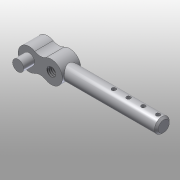
# Autodesk Inventor part: 500-178
Saved by Autodesk Inventor 2016 (Build 200138000, 138)
## iProperties
Created: 2015-04-18
Part Number: 500-178
Material: ABS Plastic
Document SubType Name: Modeling
Designer: Station9
Density: 1.06 g/cm^3
Appearance: Smooth - White
Mass: 0.63043 g
Surface Area: 6.93411 cm^2
Volume: 0.594746 cm^3
Author: Station9
Autodesk Inventor part; units mm, degrees
ref_plane "YZ Plane" through (0, 0, 0) normal (1, 0, 0) x (0, 1, 0)
ref_plane "XZ Plane" through (0, 0, 0) normal (0, 1, 0) x (-1, 0, 0)
ref_plane "XY Plane" through (0, 0, 0) normal (0, 0, 1) x (1, 0, 0)
sketch "Sketch1" plane through (0, 0, 0) normal (0, 1, 0) x (-1, 0, 0)
  arc A0 (1.5, -2.5981) -> (1.5, 2.5981) centre (3, 0) ccw
  arc A1 (-1.5, 2.5981) -> (-1.5, -2.5981) centre (-3, 0) ccw
  arc A2 (-1.5, 2.5981) -> (1.5, 2.5981) centre (0, 5.1962) ccw
  arc A3 (1.5, -2.5981) -> (-1.5, -2.5981) centre (0, -5.1962) ccw
  point P0 (0, 0)
  dimension "d0" = 6
  dimension "d1" = 6
  dimension "d2" = 6
  dimension "d3" = 3
  dimension "d4" = 6
  dimension "d5" = 6
  constraints: 8 point on circle, 4 centre point, 4 equal radius
  measures "d0" diameter of A0
  measures "d1" diameter of A1
  measures "d2" distance of A0.centre A1.centre
  measures "d3" distance of point (0, 0) A1.centre
  measures "d4" diameter of A2
  measures "d5" diameter of A3
extrude "Extrusion1" add sketch "Sketch1" along normal mid plane 5
sketch "Sketch2" plane through (0, 0, 0) normal (1, 0, 0) x (0, 1, 0)
  circle A0 centre (0, 0) radius 2
  dimension "d8" = 4
  constraints: 1 centre point, 1 coincident
  measures "d8" diameter of A0
extrude "Extrusion2" add sketch "Sketch2" along normal blind 31
sketch "Sketch3" plane through (0, -2.5, 0) normal (0, -1, 0) x (1, 0, 0)
  arc A0 (-1.5, 2.5981) -> (-1.5, -2.5981) centre (-3, 0) ccw projected
  circle A1 centre (-3, 0) radius 1.5
  point P0 (0, 0)
  dimension "d11" = 3
  constraints: 1 centre point, 1 coincident
  measures "d11" diameter of A1
extrude "Extrusion3" add sketch "Sketch3" along normal blind 3
hole "Hole1" at (3, -2.5, 0) direction (0, 1, 0) diameter 2.459 depth 8.8 tip angle 118 thread size "M3x0.5" class "6H" standard "ISO Metric profile"
sketch "Sketch4" plane through (0, 0, 0) normal (0, 0, 1) x (1, 0, 0)
  line L0 (-1.5, -2.5) -> (-1.5, -5.5) construction
  line L1 (-1.5, -5.5) -> (-4.5, -5.5) construction
  line L2 (-4.5, -5.5) -> (-4.5, -2.5) construction
  line L3 (-4.5, -2.5) -> (-6, -2.5) construction
  line L4 (-6, -2.5) -> (-6, 2.5) construction
  line L5 (-6, 2.5) -> (1.7705, 2.5) construction
  line L6 (1.7705, 2.5) -> (1.7705, -2.5) construction
  line L7 (1.7705, -2.5) -> (-1.5, -2.5) construction
  line L8 (6, 2) -> (31, 2) construction
  line L9 (31, 2) -> (31, -2) construction
  line L10 (31, -2) -> (6, -2) construction
  line L11 (6, -2) -> (6, -2.5) construction
  line L12 (6, -2.5) -> (4.2295, -2.5) construction
  line L13 (4.2295, -2.5) -> (4.2295, 2.5) construction
  line L14 (4.2295, 2.5) -> (6, 2.5) construction
  line L15 (6, 2.5) -> (6, 2) construction
  circle A0 centre (29.5, 0) radius 0.55
  point P0 (0, 0)
  dimension "d23" = 1.1
  dimension "d24" = 1.5
  constraints: 1 centre point
  measures "d23" diameter of A0
  measures "d24" distance from line of L9 A0.centre
extrude "Extrusion4" cut sketch "Sketch4" along normal mid plane 17.5
pattern_linear "Rectangular Pattern1" count 4 spacing 4 along (-1, 0, 0) of "Extrusion4"
chamfer "Chamfer1" distance 0.5 angle 45 1 edges at (31, -2, 0)
body "Solid1"
